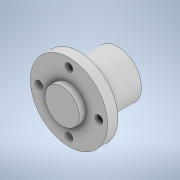
# Autodesk Inventor part: Matriz inferior do Ferramental
Saved by Autodesk Inventor 2020 (Build 240168000, 168)
## iProperties
Created: 2022-04-26
Part Number: Matriz inferior do Ferramental
Material: Genérico
Document SubType Name: Modeling
Designer: robofei
Density: 1 g/cm^3
Appearance: Padrão
Author: robofei
Autodesk Inventor part; units mm, degrees
ref_plane "YZ Plane" through (0, 0, 0) normal (1, 0, 0) x (0, 1, 0)
ref_plane "XZ Plane" through (0, 0, 0) normal (0, 1, 0) x (-1, 0, 0)
ref_plane "XY Plane" through (0, 0, 0) normal (0, 0, 1) x (1, 0, 0)
sketch "Esboço1" plane through (0, 0, 0) normal (0, 0, 1) x (1, 0, 0)
  circle A0 centre (0, 0) radius 27.5
  dimension "d0" = 55
  constraints: 1 centre point, 1 coincident
  measures "d0" diameter of A0
extrude "Extrusão1" add sketch "Esboço1" along normal blind 45
sketch "Esboço2" plane through (0, 0, 45) normal (0, 0, 1) x (1, 0, 0)
  circle A0 centre (0, 0) radius 45
  dimension "d3" = 90
  constraints: 1 centre point, 1 coincident
  measures "d3" diameter of A0
extrude "Extrusão2" add sketch "Esboço2" along normal blind 12
sketch "Esboço3" plane through (0, 0, 57) normal (0, 0, 1) x (1, 0, 0)
  circle A0 centre (35, 0) radius 4.5
  circle A1 centre (0, 35) radius 4.5
  circle A2 centre (-35, 0) radius 4.5
  circle A3 centre (0, -35) radius 4.5
  point P0 (0, 0)
  dimension "d7" = 9
  dimension "d8" = 35
  dimension "d11" = 360
  constraints: 4 centre point, 9 other
  measures "d7" diameter of A0
  measures "d8" distance of point (0, 0) A0.centre
extrude "Extrusão3" cut sketch "Esboço3" against normal blind 17.5
sketch "Esboço4" plane through (0, 0, 57) normal (0, 0, 1) x (1, 0, 0)
  circle A0 centre (0, 0) radius 27.5 projected
  circle A1 centre (0, 0) radius 20
  dimension "d15" = 40
  constraints: 1 centre point, 1 coincident
  measures "d15" diameter of A1
extrude "Extrusão4" add sketch "Esboço4" along normal blind 8 contours A1
sketch "Esboço6" plane through (0, 0, 0) normal (0, 0, -1) x (-1, 0, 0)
  line L0 (0, 10) -> (0, -10) construction
  line L1 (7.76, 10) -> (7.76, -10)
  line L2 (-7.76, -10) -> (-7.76, 10)
  arc A0 (7.76, 10) -> (-7.76, 10) centre (0, 10) ccw
  arc A1 (-7.76, -10) -> (7.76, -10) centre (0, -10) ccw
  point P0 (0, 0)
  point P1 (0, 0)
  dimension "d24" = 7.76
  dimension "d25" = 20
  dimension "d26" = 0
  dimension "d27" = 0
  constraints: 8 end point, 4 point on circle, 4 tangent, 2 centre point, 1 midpoint, 1 parallel, 1 vertical, 1 other
  measures "d24" radius of A1
  measures "d25" distance of L1.start L1.end
  measures "d26" distance of point (0, 0) point (0, 0)
  measures "d27" distance of point (0, 0) point (0, 0)
extrude "Extrusão5" cut sketch "Esboço6" against normal blind 10 draft -10
